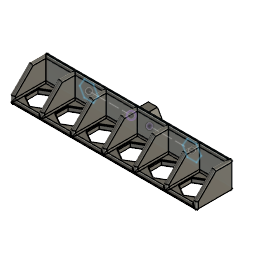
Pliers (Autodesk Fusion 360 design; units mm, degrees)
part number: 2025-05-07-10-40-20-529
Autodesk Fusion 360 part; units mm, degrees
sketch "Sketch1" plane through (0, 0, 0) normal (0, 0, 1) x (1, 0, 0)
  line L0 (75, 15) -> (-75, 15)
  line L1 (-75, 15) -> (-75, -15)
  line L2 (-75, -15) -> (75, -15)
  line L3 (75, -15) -> (75, 15)
  line L4 (75, 15) -> (-75, -15) construction
  line L5 (-75, 15) -> (75, -15) construction
  dimension "d1" = 150
  dimension "d2" = 30
  constraint horizontal L0
  constraint perpendicular L0 L1
  constraint parallel L0 L2
  constraint parallel L1 L3
  constraint coincident L4 origin
  constraint coincident L5 origin
  measures "d1" distance of L1.end L2.end
  measures "d2" distance of L0.end L1.end
extrude "Extrude1" add sketch "Sketch1" along normal blind 4
sketch "Sketch2" plane through (0, 0, 4) normal (0, 0, 1) x (-1, 0, 0)
  line L0 (-75, 15) -> (-75, -15)
  line L1 (-75, -15) -> (75, -15)
  line L2 (75, -15) -> (75, 15)
  line L3 (75, 15) -> (-75, 15)
  line L4 (75, -15) -> (-75, -15)
  line L5 (-75, -15) -> (-75, -11)
  line L6 (-75, -11) -> (75, -11)
  line L7 (75, -11) -> (75, -15)
  dimension "d5" = 4
  constraint horizontal L4
  constraint vertical L5
  constraint horizontal L6
  constraint vertical L7
  constraint coincident L1.end L2.start
  measures "d5" distance of L1.end L6.end
extrude "Extrude2" add sketch "Sketch2" along normal blind 21 contours L0 L1 L2 L4 L5 L6 L7
sketch "Sketch3" plane through (0, 0, 4) normal (0, 0, 1) x (-1, 0, 0)
  line L0 (-75, -11) -> (75, -11)
  line L1 (75, -11) -> (75, 15)
  line L2 (75, 15) -> (-75, 15)
  line L3 (-75, 15) -> (-75, -11)
  line L4 (75, 15) -> (72, 15)
  line L5 (72, 15) -> (72, -11)
  line L6 (72, -11) -> (75, -11)
  line L7 (75, -11) -> (75, 15)
  line L8 (51.5, 15) -> (48.5, 15)
  line L9 (48.5, 15) -> (48.5, -11)
  line L10 (48.5, -11) -> (51.5, -11)
  line L11 (51.5, -11) -> (51.5, 15)
  line L12 (26.5, 15) -> (23.5, 15)
  line L13 (23.5, 15) -> (23.5, -11)
  line L14 (23.5, -11) -> (26.5, -11)
  line L15 (26.5, -11) -> (26.5, 15)
  line L16 (-75, 15) -> (-72, 15)
  line L17 (-72, 15) -> (-72, -11)
  line L18 (-72, -11) -> (-75, -11)
  line L19 (-75, -11) -> (-75, 15)
  line L20 (-51.5, 15) -> (-48.5, 15)
  line L21 (-48.5, 15) -> (-48.5, -11)
  line L22 (-48.5, -11) -> (-51.5, -11)
  line L23 (-51.5, -11) -> (-51.5, 15)
  line L24 (-26.5, 15) -> (-23.5, 15)
  line L25 (-23.5, 15) -> (-23.5, -11)
  line L26 (-23.5, -11) -> (-26.5, -11)
  line L27 (-26.5, -11) -> (-26.5, 15)
  line L28 (-1.5173, 15) -> (1.4827, 15)
  line L29 (1.4827, 15) -> (1.4827, -11)
  line L30 (1.4827, -11) -> (-1.5173, -11)
  line L31 (-1.5173, -11) -> (-1.5173, 15)
  dimension "d8" = 3
  dimension "d9" = 3
  dimension "d10" = 3
  dimension "d11" = 3
  dimension "d12" = 3
  dimension "d13" = 3
  dimension "d15" = 3
  constraint horizontal L4
  constraint vertical L5
  constraint horizontal L6
  constraint vertical L7
  constraint coincident L1.end L2.start
  constraint horizontal L8
  constraint vertical L9
  constraint horizontal L10
  constraint vertical L11
  constraint coincident L2 L8.start
  constraint horizontal L12
  constraint vertical L13
  constraint horizontal L14
  constraint vertical L15
  constraint coincident L2 L12.start
  constraint horizontal L16
  constraint vertical L17
  constraint horizontal L18
  constraint vertical L19
  constraint coincident L2.end L3.start
  constraint horizontal L20
  constraint vertical L21
  constraint horizontal L22
  constraint vertical L23
  constraint coincident L2 L20.start
  constraint horizontal L24
  constraint vertical L25
  constraint horizontal L26
  constraint vertical L27
  constraint coincident L2 L24.start
  constraint horizontal L28
  constraint vertical L29
  constraint horizontal L30
  constraint vertical L31
  constraint coincident L2 L28.start
  measures "d8" distance of L1.end L4.end
  measures "d9" distance of L8.start L8.end
  measures "d10" distance of L12.start L12.end
  measures "d11" distance of L2.end L16.end
  measures "d12" distance of L20.start L20.end
  measures "d13" distance of L24.start L24.end
  measures "d15" distance of L28.start L28.end
extrude "Extrude3" add sketch "Sketch3" along normal blind 18 contours L0 L2 L3 L16 L17 L18 L19 | L0 L2 L20 L21 L22 L23 | L0 L2 L24 L25 L26 L27 | L0 L2 L28 L29 L30 L31 | L0 L2 L12 L13 L14 L15 | L0 L2 L8 L9 L10 L11 | L0 L1 L2 L4 L5 L6 L7
extrude "Extrude4" cut 1 faces at (-25, 13.6667, 25) along direction (0, 0, -1) blind 3
chamfer "Chamfer1" distance 15 angle 45 7 edges at (-73.5, -15, 22) (-50, -15, 22) (-25, -15, 22) (0.0173, -15, 22) (25, -15, 22) (50, -15, 22) (73.5, -15, 22)
sketch "Sketch4" plane through (0, 0, 4) normal (0, 0, 1) x (-1, 0, 0)
  line L0 (23.5, -11) -> (23.5, 15)
  line L1 (23.5, 15) -> (1.4827, 15)
  line L2 (1.4827, 15) -> (1.4827, -11)
  line L3 (1.4827, -11) -> (23.5, -11)
  line L4 (12.4914, -8) -> (21.1516, -3)
  line L5 (21.1516, -3) -> (21.1516, 7)
  line L6 (21.1516, 7) -> (12.4914, 12)
  line L7 (12.4914, 12) -> (3.8311, 7)
  line L8 (3.8311, 7) -> (3.8311, -3)
  line L9 (3.8311, -3) -> (12.4914, -8)
  point P0 (12.4914, 2)
  dimension "d21" = 10
  measures "d21" distance of L4.start P0
extrude "Extrude5" cut sketch "Sketch4" against normal up to surface (4 mm away) contours L4 L5 L6 L7 L8 L9
sketch "Sketch5" plane through (0, 0, 4) normal (0, 0, 1) x (-1, 0, 0)
  line L0 (26.5, 15) -> (26.5, -11)
  line L1 (26.5, -11) -> (48.5, -11)
  line L2 (48.5, -11) -> (48.5, 15)
  line L3 (48.5, 15) -> (26.5, 15)
  line L4 (26.5, 2) -> (48.5, 2) construction
  line L5 (37.5, 12) -> (28.8397, 7)
  line L6 (28.8397, 7) -> (28.8397, -3)
  line L7 (28.8397, -3) -> (37.5, -8)
  line L8 (37.5, -8) -> (46.1603, -3)
  line L9 (46.1603, -3) -> (46.1603, 7)
  line L10 (46.1603, 7) -> (37.5, 12)
  point P0 (37.5, 2)
  dimension "d24" = 10
  constraint midpoint L0 L4.start
  constraint midpoint L2 L4.end
  constraint midpoint L4 P0
  measures "d24" distance of L5.start P0
extrude "Extrude6" cut sketch "Sketch5" against normal up to surface (4 mm away) contours L5 L6 L7 L8 L9 L10
sketch "Sketch6" plane through (0, 0, 4) normal (0, 0, 1) x (-1, 0, 0)
  line L0 (51.5, 15) -> (51.5, -11)
  line L1 (51.5, -11) -> (72, -11)
  line L2 (72, -11) -> (72, 15)
  line L3 (72, 15) -> (51.5, 15)
  line L4 (51.5, 2) -> (72, 2) construction
  line L5 (61.75, 12) -> (53.0897, 7)
  line L6 (53.0897, 7) -> (53.0897, -3)
  line L7 (53.0897, -3) -> (61.75, -8)
  line L8 (61.75, -8) -> (70.4103, -3)
  line L9 (70.4103, -3) -> (70.4103, 7)
  line L10 (70.4103, 7) -> (61.75, 12)
  point P0 (61.75, 2)
  dimension "d27" = 10
  constraint midpoint L0 L4.start
  constraint midpoint L2 L4.end
  constraint midpoint L4 P0
  measures "d27" distance of L5.start P0
extrude "Extrude7" cut sketch "Sketch6" against normal up to surface (4 mm away) contours L5 L6 L7 L8 L9 L10
sketch "Sketch7" plane through (0, 0, 4) normal (0, 0, 1) x (-1, 0, 0)
  line L0 (-1.5173, -11) -> (-1.5173, 15)
  line L1 (-1.5173, 15) -> (-23.5, 15)
  line L2 (-23.5, 15) -> (-23.5, -11)
  line L3 (-23.5, -11) -> (-1.5173, -11)
  line L4 (-23.5, 2) -> (-1.5173, 2) construction
  line L5 (-12.5086, 15) -> (-12.5086, -11) construction
  line L6 (-12.5086, 12) -> (-21.1689, 7)
  line L7 (-21.1689, 7) -> (-21.1689, -3)
  line L8 (-21.1689, -3) -> (-12.5086, -8)
  line L9 (-12.5086, -8) -> (-3.8484, -3)
  line L10 (-3.8484, -3) -> (-3.8484, 7)
  line L11 (-3.8484, 7) -> (-12.5086, 12)
  point P0 (-12.5086, 2)
  dimension "d30" = 10
  constraint midpoint L2 L4.start
  constraint midpoint L0 L4.end
  constraint midpoint L1 L5.start
  constraint midpoint L3 L5.end
  constraint coincident L5 L6.start
  constraint midpoint L5 P0
  measures "d30" distance of L6.start P0
extrude "Extrude8" cut sketch "Sketch7" against normal up to surface (4 mm away) contours L6 L7 L8 L9 L10 L11
sketch "Sketch8" plane through (0, 0, 4) normal (0, 0, 1) x (-1, 0, 0)
  line L0 (-48.5, 15) -> (-48.5, -11)
  line L1 (-48.5, -11) -> (-26.5, -11)
  line L2 (-26.5, -11) -> (-26.5, 15)
  line L3 (-26.5, 15) -> (-48.5, 15)
  line L4 (-26.5, 2) -> (-48.5, 2) construction
  line L5 (-37.5, 15) -> (-37.5, -11) construction
  line L6 (-37.5, 12) -> (-46.1603, 7)
  line L7 (-46.1603, 7) -> (-46.1603, -3)
  line L8 (-46.1603, -3) -> (-37.5, -8)
  line L9 (-37.5, -8) -> (-28.8397, -3)
  line L10 (-28.8397, -3) -> (-28.8397, 7)
  line L11 (-28.8397, 7) -> (-37.5, 12)
  point P0 (-37.5, 2)
  dimension "d33" = 10
  constraint midpoint L2 L4.start
  constraint midpoint L0 L4.end
  constraint midpoint L3 L5.start
  constraint midpoint L1 L5.end
  constraint coincident L5 L6.start
  constraint midpoint L5 P0
  measures "d33" distance of L6.start P0
extrude "Extrude9" cut sketch "Sketch8" against normal up to surface (4 mm away) contours L6 L7 L8 L9 L10 L11
sketch "Sketch9" plane through (0, 0, 4) normal (0, 0, 1) x (-1, 0, 0)
  line L0 (-72, 15) -> (-72, -11)
  line L1 (-72, -11) -> (-51.5, -11)
  line L2 (-51.5, -11) -> (-51.5, 15)
  line L3 (-51.5, 15) -> (-72, 15)
  line L4 (-61.75, 15) -> (-61.75, -11) construction
  line L5 (-51.5, 2) -> (-72, 2) construction
  line L6 (-61.75, 12) -> (-70.4103, 7)
  line L7 (-70.4103, 7) -> (-70.4103, -3)
  line L8 (-70.4103, -3) -> (-61.75, -8)
  line L9 (-61.75, -8) -> (-53.0897, -3)
  line L10 (-53.0897, -3) -> (-53.0897, 7)
  line L11 (-53.0897, 7) -> (-61.75, 12)
  point P0 (-61.75, 2)
  dimension "d36" = 10
  constraint midpoint L3 L4.start
  constraint midpoint L1 L4.end
  constraint midpoint L2 L5.start
  constraint midpoint L0 L5.end
  constraint midpoint L5 P0
  constraint coincident L4 L6.start
  measures "d36" distance of L6.start P0
extrude "Extrude10" cut sketch "Sketch9" against normal up to surface (4 mm away) contours L6 L7 L8 L9 L10 L11
fillet "Fillet1" radius 1.5 54 edges at (-75, -7.5, 14.5) (-75, 7.5, 22) (-75, -15, 3.5) (-72, 5.5, 22) (-72, -7.5, 14.5) (-72, -15, 5.5) (-51.5, 5.5, 22) (-51.5, -7.5, 14.5) (-51.5, -15, 5.5) (-48.5, 5.5, 22) (-48.5, -7.5, 14.5) (-48.5, -15, 5.5) (-26.5, 5.5, 22) (-26.5, -7.5, 14.5) (-26.5, -15, 5.5) (-23.5, 5.5, 22) (-23.5, -7.5, 14.5) (-23.5, -15, 5.5) (-1.4827, 5.5, 22) (-1.4827, -7.5, 14.5) (-1.4827, -15, 5.5) (1.5173, 5.5, 22) (1.5173, -7.5, 14.5) (1.5173, -15, 5.5) (23.5, 5.5, 22) (23.5, -7.5, 14.5) (23.5, -15, 5.5) (26.5, 5.5, 22) (26.5, -7.5, 14.5) (26.5, -15, 5.5) (48.5, 5.5, 22) (48.5, -7.5, 14.5) (48.5, -15, 5.5) (51.5, 5.5, 22) (51.5, -7.5, 14.5) (51.5, -15, 5.5) (72, 5.5, 22) (72, -7.5, 14.5) (72, -15, 5.5) (75, 7.5, 22) (75, -7.5, 14.5) (75, -15, 3.5) (61.75, 11, 22) (37.5, 11, 22) (12.5086, 11, 22) (-12.4914, 11, 22) (-37.5, 11, 22) (-61.75, 11, 22) (-61.75, -15, 4) (-37.5, -15, 4) (-12.4914, -15, 4) (12.5086, -15, 4) (37.5, -15, 4) (61.75, -15, 4)
fillet "Fillet2" radius 1.5 6 edges at (-75, 15, 10.25) (-74.5607, 15, 21.5607) (0, 15, 22) (74.5607, 15, 21.5607) (75, 15, 10.25) (0, 15, 0)
fillet "Fillet3" radius 1.5 7 edges at (-74.5607, 14.5607, 0.4393) (-75, 0, 0) (-74.5607, -14.5607, 0) (0, -15, 0) (74.5607, -14.5607, 0) (75, 0, 0) (74.5607, 14.5607, 0.4393)
fillet "Fillet4" radius 1 30 edges at (-72, -1.25, 4) (-72.4393, -14.5607, 3.5607) (-61.75, 11, 4) (-51.0607, -14.5607, 3.5607) (-51.5, -1.25, 4) (-48.5, -1.25, 4) (-48.9393, -14.5607, 3.5607) (-37.5, 11, 4) (-26.0607, -14.5607, 3.5607) (-26.5, -1.25, 4) (-23.5, -1.25, 4) (-23.9393, -14.5607, 3.5607) (-12.4914, 11, 4) (-1.0434, -14.5607, 3.5607) (-1.4827, -1.25, 4) (1.5173, -1.25, 4) (1.0779, -14.5607, 3.5607) (12.5086, 11, 4) (23.9393, -14.5607, 3.5607) (23.5, -1.25, 4) (26.5, -1.25, 4) (26.0607, -14.5607, 3.5607) (37.5, 11, 4) (48.9393, -14.5607, 3.5607) (48.5, -1.25, 4) (51.5, -1.25, 4) (51.0607, -14.5607, 3.5607) (61.75, 11, 4) (72.4393, -14.5607, 3.5607) (72, -1.25, 4)
chamfer "Chamfer2" distance 0.5 angle 45 6 edges at (-70.4103, -2, 4) (-66.0801, 5.5, 4) (-57.4199, 5.5, 4) (-57.4199, -9.5, 4) (-66.0801, -9.5, 4) (-53.0897, -2, 4)
chamfer "Chamfer3" distance 0.5 angle 45 30 edges at (-41.8301, 5.5, 4) (-33.1699, 5.5, 4) (-46.1603, -2, 4) (-41.8301, -9.5, 4) (-28.8397, -2, 4) (-33.1699, -9.5, 4) (-16.8215, 5.5, 4) (-21.1516, -2, 4) (-16.8215, -9.5, 4) (-8.1612, 5.5, 4) (-3.8311, -2, 4) (-8.1612, -9.5, 4) (3.8484, -2, 4) (8.1785, 5.5, 4) (16.8388, 5.5, 4) (21.1689, -2, 4) (16.8388, -9.5, 4) (8.1785, -9.5, 4) (28.8397, -2, 4) (33.1699, 5.5, 4) (41.8301, 5.5, 4) (46.1603, -2, 4) (41.8301, -9.5, 4) (33.1699, -9.5, 4) (53.0897, -2, 4) (57.4199, 5.5, 4) (66.0801, 5.5, 4) (70.4103, -2, 4) (66.0801, -9.5, 4) (57.4199, -9.5, 4)
chamfer "Chamfer4" distance 0.5 angle 45 36 edges at (-66.0801, -9.5, 0) (-57.4199, -9.5, 0) (-53.0897, -2, 0) (-57.4199, 5.5, 0) (-66.0801, 5.5, 0) (-70.4103, -2, 0) (-41.8301, -9.5, 0) (-46.1603, -2, 0) (-41.8301, 5.5, 0) (-33.1699, -9.5, 0) (-28.8397, -2, 0) (-33.1699, 5.5, 0) (-16.8215, -9.5, 0) (-21.1516, -2, 0) (-16.8215, 5.5, 0) (-8.1612, -9.5, 0) (-8.1612, 5.5, 0) (-3.8311, -2, 0) (3.8484, -2, 0) (8.1785, -9.5, 0) (16.8388, -9.5, 0) (8.1785, 5.5, 0) (16.8388, 5.5, 0) (21.1689, -2, 0) (28.8397, -2, 0) (33.1699, -9.5, 0) (41.8301, -9.5, 0) (46.1603, -2, 0) (41.8301, 5.5, 0) (33.1699, 5.5, 0) (57.4199, -9.5, 0) (66.0801, -9.5, 0) (70.4103, -2, 0) (66.0801, 5.5, 0) (57.4199, 5.5, 0) (53.0897, -2, 0)
sketch "Sketch10" plane through (0, 15, 0) normal (0, 1, 0) x (-1, 0, 0)
  line L0 (-73.5, 1.5) -> (73.5, 1.5)
  line L1 (73.5, 1.5) -> (73.5, 20.5)
  line L2 (73.5, 20.5) -> (-73.5, 20.5)
  line L3 (-73.5, 20.5) -> (-73.5, 1.5)
  line L4 (-73.5, 11) -> (73.5, 11) construction
  line L5 (7.4, 11) -> (3.7, 17.4086)
  line L6 (3.7, 17.4086) -> (-3.7, 17.4086)
  line L7 (-3.7, 17.4086) -> (-7.4, 11)
  line L8 (-7.4, 11) -> (-3.7, 4.5914)
  line L9 (-3.7, 4.5914) -> (3.7, 4.5914)
  line L10 (3.7, 4.5914) -> (7.4, 11)
  point P0 (0, 11)
  dimension "d50" = 7.4
  constraint midpoint L3 L4.start
  constraint midpoint L1 L4.end
  constraint midpoint L4 P0
  measures "d50" distance of L5.start P0
extrude "Extrude11" add sketch "Sketch10" along normal blind 10 contours L5 L6 L7 L8 L9 L10
sketch "Sketch11" plane through (0, 15, 0) normal (0, 1, 0) x (-1, 0, 0)
  line L0 (3.7, 4.5914) -> (-3.7, 4.5914)
  line L1 (-3.7, 4.5914) -> (-7.4, 11)
  line L2 (-7.4, 11) -> (-3.7, 17.4086)
  line L3 (-3.7, 17.4086) -> (3.7, 17.4086)
  line L4 (3.7, 17.4086) -> (7.4, 11)
  line L5 (7.4, 11) -> (3.7, 4.5914)
  line L6 (-73.5, 1.5) -> (73.5, 1.5)
  line L7 (73.5, 1.5) -> (73.5, 20.5)
  line L8 (73.5, 20.5) -> (-73.5, 20.5)
  line L9 (-73.5, 20.5) -> (-73.5, 1.5)
  line L10 (7.4, 11) -> (34, 11) construction
  line L11 (34, 11) -> (41.4, 11) construction
  line L12 (48.8, 11) -> (45.1, 17.4086)
  line L13 (45.1, 17.4086) -> (37.7, 17.4086)
  line L14 (37.7, 17.4086) -> (34, 11)
  line L15 (34, 11) -> (37.7, 4.5914)
  line L16 (37.7, 4.5914) -> (45.1, 4.5914)
  line L17 (45.1, 4.5914) -> (48.8, 11)
  line L18 (-7.4, 11) -> (-41.4, 11) construction
  line L19 (-34, 11) -> (-37.7, 17.4086)
  line L20 (-37.7, 17.4086) -> (-45.1, 17.4086)
  line L21 (-45.1, 17.4086) -> (-48.8, 11)
  line L22 (-48.8, 11) -> (-45.1, 4.5914)
  line L23 (-45.1, 4.5914) -> (-37.7, 4.5914)
  line L24 (-37.7, 4.5914) -> (-34, 11)
  point P0 (7.4, 11)
  point P1 (-7.4, 11)
  point P2 (41.4, 11)
  point P3 (-41.4, 11)
  dimension "d53" = 26.6
  dimension "d54" = 14.8
  dimension "d55" = 7.4
  dimension "d56" = 7.4
  dimension "d57" = 34
  dimension "d58" = 7.4
  constraint coincident P0 L4.end
  constraint parallel L6 L10
  constraint parallel L10 L11
  constraint coincident P2 L11.end
  constraint coincident P1 L1.end
  constraint parallel L6 L18
  constraint coincident P3 L18.end
  measures "d53" distance of P0 L10.end
  measures "d54" distance of P0 P1
  measures "d55" distance of L10.end P2
  measures "d56" distance of L12.start P2
  measures "d57" distance of P1 P3
  measures "d58" distance of L19.start P3
extrude "Extrude12" [suppressed]
chamfer "Chamfer5" [suppressed]
fillet "Fillet5" [suppressed]
equation "d1 = ( 25 * 6 ) * 1 mm"
equation "d6 = 25 mm - 4 mm"
equation "d55 = ( 14.8 / 2 ) * 1 mm"
equation "d57 = 26.6 mm + 7.4 mm"
